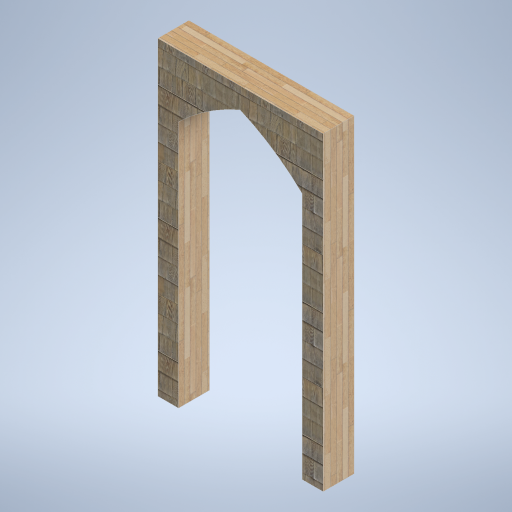
# Autodesk Inventor part: front_wall_block06
Saved by Autodesk Inventor 2024.2 (Build 282272000, 272)
## iProperties
Created: 2024-05-23
Part Number: front_wall_block06
Material: Wood (Maple)
Document SubType Name: Modeling
Designer: LOSTER_1
Density: 0.67 g/cm^3
Appearance: Natural Maple - Glossy Dark Tint
Author: LOSTER_1
Autodesk Inventor part; units mm, degrees
ref_plane "YZ Plane" through (0, 0, 0) normal (1, 0, 0) x (0, 1, 0)
ref_plane "XZ Plane" through (0, 0, 0) normal (0, 1, 0) x (-1, 0, 0)
ref_plane "XY Plane" through (0, 0, 0) normal (0, 0, 1) x (1, 0, 0)
sketch "Sketch1" plane through (0, 0, 0) normal (0, 0, 1) x (1, 0, 0)
  line L0 (-797.6302, 1502.3971) -> (802.3698, 1502.3971)
  line L1 (-797.6302, -1497.6029) -> (-797.6302, 1502.3971)
  line L2 (802.3698, -1497.6029) -> (802.3698, 1502.3971)
  line L3 (-797.6302, -1497.6029) -> (802.3698, -1497.6029)
  point P0 (0, 0)
  constraints: 8 end point, 1 horizontal
extrude "Extrusion1" add sketch "Sketch1" along normal blind 300
sketch "Sketch2" plane through (0, 0, 300) normal (0, 0, 1) x (1, 0, 0)
  line L0 (2.3698, -1497.6029) -> (-2.3622, -1497.6029)
  line L1 (-797.6302, -1495.094) -> (-807.0903, -1495.0642)
  line L2 (-597.6243, 900.5193) -> (-597.6243, -1497.6029)
  line L3 (-597.6243, -1497.6029) -> (-597.6243, 902.3971)
  line L4 (597.6243, 900.5193) -> (597.6243, -1497.6029)
  line L5 (-597.6243, -1497.6029) -> (597.6243, -1497.6029)
  arc A0 (-2.0612, 1300.518) -> (-597.6243, 902.3971) centre (793.6714, -534.3687) ccw
  arc A1 (597.6243, 900.5193) -> (-2.0612, 1300.518) centre (-793.8493, -536.0744) ccw
  point P0 (0, 0)
  point P1 (2.0612, 1300.518)
  dimension "d8" = 2000
  dimension "d9" = 2000
  constraints: 12 end point, 4 point on circle, 2 centre point, 2 point on line, 1 perpendicular
  measures "d8" radius of A0
  measures "d9" radius of A1
extrude "Extrusion2" cut sketch "Sketch2" against normal through all
body "Solid1"
